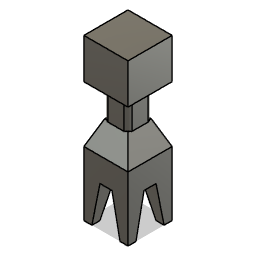
NovoCreeperV3 v1 (Autodesk Fusion 360 design; units mm, degrees)
Autodesk Fusion 360 part; units mm, degrees
sketch "Esboço1" plane through (0, 0, 0) normal (0, 1, 0) x (1, 0, 0)
  line L0 (0, 0) -> (55, 0)
  line L1 (55, 0) -> (55, -55)
  line L2 (55, -55) -> (0, -55)
  line L3 (0, -55) -> (0, 0)
  dimension "d1" = 55
  dimension "d2" = 55
  constraint horizontal L0
  constraint vertical L1
  constraint horizontal L2
  constraint vertical L3
  constraint coincident L0.start L3.end
  measures "d1" distance of L0.start L0.end
  measures "d2" distance of L0.start L2.end
extrude "Extrusão1" add sketch "Esboço1" along normal blind 200
sketch "Esboço2" plane through (0, 0, 55) normal (0, 0, 1) x (1, 0, 0)
  line L0 (0, 0) -> (55, 0)
  line L1 (55, 0) -> (55, 200)
  line L2 (55, 200) -> (0, 200)
  line L3 (0, 200) -> (0, 0)
  line L4 (0, 110) -> (12.5, 110)
  line L5 (12.5, 110) -> (12.5, 150)
  line L6 (12.5, 150) -> (0, 150)
  line L7 (0, 150) -> (0, 110)
  dimension "d5" = 12.5
  dimension "d6" = 40
  constraint horizontal L4
  constraint vertical L5
  constraint horizontal L6
  constraint vertical L7
  constraint coincident L3 L4.start
  measures "d5" distance of L4.start L4.end
  measures "d6" distance of L4.start L6.end
extrude "Extrusão2" cut sketch "Esboço2" against normal blind 80 contours L3 L4 L5 L6 L7
sketch "Esboço3" plane through (0, 0, 55) normal (0, 0, 1) x (1, 0, 0)
  line L0 (12.5, 110) -> (0, 110)
  line L1 (0, 110) -> (0, 0)
  line L2 (0, 0) -> (55, 0)
  line L3 (55, 0) -> (55, 200)
  line L4 (55, 200) -> (0, 200)
  line L5 (0, 200) -> (0, 150)
  line L6 (0, 150) -> (12.5, 150)
  line L7 (12.5, 150) -> (12.5, 110)
  line L8 (55, 110) -> (42.5, 110)
  line L9 (42.5, 110) -> (42.5, 150)
  line L10 (42.5, 150) -> (55, 150)
  line L11 (55, 150) -> (55, 110)
  dimension "d9" = 12.5
  dimension "d10" = 40
  constraint horizontal L8
  constraint vertical L9
  constraint horizontal L10
  constraint vertical L11
  constraint coincident L3 L8.start
  measures "d9" distance of L8.start L8.end
  measures "d10" distance of L8.start L10.end
extrude "Extrusão3" cut sketch "Esboço3" against normal blind 105 contours L3 L8 L9 L10 L11
sketch "Esboço4" plane through (42.5, 0, 0) normal (1, 0, 0) x (0, 0, -1)
  line L0 (0, 110) -> (0, 150)
  line L1 (0, 150) -> (-55, 150)
  line L2 (-55, 150) -> (-55, 110)
  line L3 (-55, 110) -> (0, 110)
  line L4 (-55, 110) -> (-42.5, 110)
  line L5 (-42.5, 110) -> (-42.5, 150)
  line L6 (-42.5, 150) -> (-55, 150)
  line L7 (-55, 150) -> (-55, 110)
  dimension "d13" = 12.5
  dimension "d14" = 40
  constraint horizontal L4
  constraint vertical L5
  constraint horizontal L6
  constraint vertical L7
  constraint coincident L2.end L3.start
  measures "d13" distance of L2.end L4.end
  measures "d14" distance of L2.end L1.end
extrude "Extrusão4" cut sketch "Esboço4" against normal blind 70 contours L1 L2 L3 L4 L5 L6 L7
sketch "Esboço5" plane through (42.5, 0, 0) normal (1, 0, 0) x (0, 0, -1)
  line L0 (-42.5, 150) -> (-42.5, 110)
  line L1 (-42.5, 110) -> (0, 110)
  line L2 (0, 110) -> (0, 150)
  line L3 (0, 150) -> (-42.5, 150)
  line L4 (0, 110) -> (-12.5, 110)
  line L5 (-12.5, 110) -> (-12.5, 150)
  line L6 (-12.5, 150) -> (0, 150)
  line L7 (0, 150) -> (0, 110)
  dimension "d17" = 12.5
  dimension "d18" = 40
  constraint horizontal L4
  constraint vertical L5
  constraint horizontal L6
  constraint vertical L7
  constraint coincident L1.end L2.start
  measures "d17" distance of L1.end L4.end
  measures "d18" distance of L1.end L2.end
extrude "Extrusão5" cut sketch "Esboço5" against normal blind 60 contours L1 L2 L3 L4 L5 L6 L7
fillet "Arredondamento1" radius 5 4 edges at (42.5, 130, 12.5) (12.5, 130, 12.5) (42.5, 130, 42.5) (12.5, 130, 42.5)
sketch "Esboço6" plane through (55, 0, 0) normal (1, 0, 0) x (0, 0, -1)
  line L0 (0, 110) -> (-55, 110)
  line L1 (-55, 110) -> (-55, 0)
  line L2 (-55, 0) -> (0, 0)
  line L3 (0, 0) -> (0, 110)
  line L4 (-45, 0) -> (-35, 50)
  line L5 (-35, 50) -> (-20, 50)
  line L6 (-20, 50) -> (-10, 0)
  line L7 (-45, 0) -> (-10, 0)
  dimension "d23" = 10
  constraint coincident L2 L4.start
  constraint perpendicular L3 L5
  constraint coincident L2 L6.end
  measures "d23" distance of L1.end L4.start
extrude "Extrusão6" cut sketch "Esboço6" against normal blind 120 contours L2 L4 L5 L6 L7
sketch "Esboço7" plane through (0, 0, 0) normal (0, 0, -1) x (-1, 0, 0)
  line L0 (0, 110) -> (-55, 110)
  line L1 (-55, 110) -> (-55, 0)
  line L2 (-55, 0) -> (0, 0)
  line L3 (0, 0) -> (0, 110)
  line L4 (-45, 0) -> (-35, 50)
  line L5 (-35, 50) -> (-20, 50)
  line L6 (-20, 50) -> (-10, 0)
  dimension "d26" = 10
  dimension "d27" = 10
  measures "d26" distance of L1.end L4.start
  measures "d27" distance of L2.end L6.end
extrude "Extrusão7" cut sketch "Esboço7" against normal blind 100 contours L2 L4 L5 L6
chamfer "Chanfro1" distance 30 distance2 13 4 edges at (27.5, 110, 0) (0, 110, 27.5) (27.5, 110, 55) (55, 110, 27.5) measured on face at (34.1667, 90, 0) measured on face at (0, 90, 30) measured on face at (34.1667, 90, 55) measured on face at (55, 90, 30)
